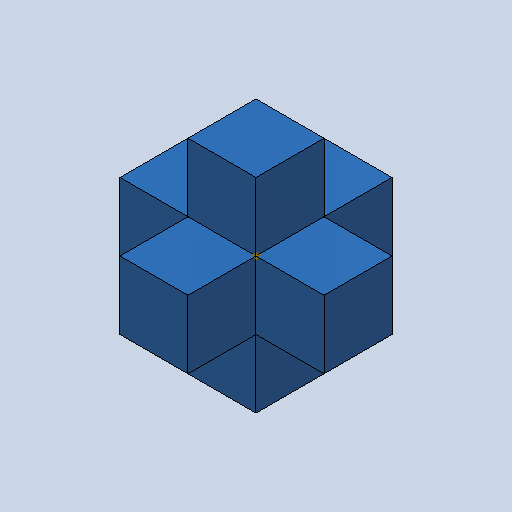
# Autodesk Inventor part: Wire termination point.0010
Saved by Autodesk Inventor 2022 (Build 260153000, 153)
## iProperties
Created: 2016-02-02
Material: Generic
Document SubType Name: Modeling
Designer: Ryan
Density: 1 g/cm^3
Appearance: Cyan
Stock Number: Cut shield at jacket
GlobalPropertyList: <PropertyList/>
Scrubbed Status: Scrubbed
Author: Ryan
Autodesk Inventor part; units mm, degrees
ref_plane "YZ Plane" through (0, 0, 0) normal (1, 0, 0) x (0, 1, 0)
ref_plane "XZ Plane" through (0, 0, 0) normal (0, 1, 0) x (-1, 0, 0)
ref_plane "XY Plane" through (0, 0, 0) normal (0, 0, 1) x (1, 0, 0)
sketch "Sketch4" plane through (0, 0, 0) normal (1, 0, 0) x (0, 1, 0)
  line L0 (0.7937, 0) -> (1.5875, 0)
  line L1 (1.5875, 0) -> (1.5875, -0.7937)
  line L2 (1.5875, -0.7937) -> (2.3813, -0.7937)
  line L3 (2.3813, -0.7937) -> (2.3813, -1.5875)
  line L4 (2.3813, -1.5875) -> (1.5875, -1.5875)
  line L5 (1.5875, -2.3812) -> (0.7938, -2.3812)
  line L6 (0.7938, -2.3812) -> (0.7938, -1.5875)
  line L7 (0.7938, -1.5875) -> (0, -1.5875)
  line L8 (0, -1.5875) -> (0, -0.7937)
  line L9 (0, -0.7937) -> (0.7938, -0.7937)
  line L10 (0.7938, -0.7937) -> (0.7937, 0)
  line L11 (1.5875, -2.3812) -> (1.5875, -1.5875)
  point P0 (0, 0)
  dimension "d16" = 0.7937
  dimension "d17" = 0.7937
  dimension "d18" = 0.7937
  dimension "d19" = 0.7937
  dimension "d20" = 0.7937
  dimension "d22" = 0.7937
  constraints: 24 end point, 8 perpendicular, 4 collinear, 4 point on line, 2 horizontal, 1 vertical
  measures "d16" distance of L0.start L0.end
  measures "d17" distance of L0.end L1.end
  measures "d18" distance of L1.end L2.end
  measures "d19" distance of L2.end L3.end
  measures "d20" distance between parallel lines of L10 L8
  measures "d22" distance between parallel lines of L5 L4
extrude "Extrusion4" add sketch "Sketch4" along normal blind 0.7937
sketch "Sketch5" plane through (0.7937, 0, 0) normal (1, 0, 0) x (0, 0, -1)
  line L0 (1.5875, 0.7938) -> (0.7937, 0.7938)
  line L1 (0.7937, 0.7938) -> (0.7937, 1.5875)
  line L2 (0.7937, 1.5875) -> (1.5875, 1.5875)
  line L3 (1.5875, 1.5875) -> (1.5875, 0.7938)
  point P0 (0, 0)
  constraints: 8 end point, 2 parallel, 1 horizontal, 1 perpendicular
extrude "Extrusion5" add sketch "Sketch5" along normal blind 0.7937
sketch "Sketch6" plane through (0, 0, 0) normal (-1, 0, 0) x (0, 0, 1)
  line L0 (-1.5875, 1.5875) -> (-0.7937, 1.5875)
  line L1 (-0.7937, 1.5875) -> (-0.7937, 0.7938)
  line L2 (-0.7937, 0.7938) -> (-1.5875, 0.7938)
  line L3 (-1.5875, 0.7938) -> (-1.5875, 1.5875)
  point P0 (0, 0)
  constraints: 8 end point, 2 parallel, 1 horizontal, 1 perpendicular
extrude "Extrusion6" add sketch "Sketch6" along normal blind 0.7937
body "Solid2"
